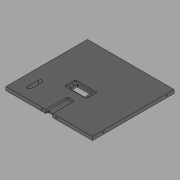
# Autodesk Inventor part: box_shelf
Saved by Autodesk Inventor 2019 (Build 230136000, 136)
## iProperties
Part Number: box_shelf
Material: Generic
Document SubType Name: Modeling
Designer: Javi
Appearance: Default
screws: 0,400 cm
Author: Javi
Autodesk Inventor part; units mm, degrees
ref_plane "YZ Plane" through (0, 0, 0) normal (1, 0, 0) x (0, 1, 0)
ref_plane "XZ Plane" through (0, 0, 0) normal (0, 1, 0) x (-1, 0, 0)
ref_plane "XY Plane" through (0, 0, 0) normal (0, 0, 1) x (1, 0, 0)
sketch "Sketch1" plane through (0, 0, 0) normal (0, 1, 0) x (-1, 0, 0)
  line L0 (0, 0) -> (-120, 0)
  line L1 (-120, 0) -> (-120, -226)
  line L2 (-120, -226) -> (0, -226)
  line L3 (0, -226) -> (0, 0)
  dimension "d0" = 120
  dimension "d1" = 226
  constraints: 8 end point, 2 parallel, 1 horizontal, 1 perpendicular
  measures "d0" distance of L2.end L1.end
  measures "d1" distance of L1.end L0.end
extrude "Extrusion1" add sketch "Sketch1" along normal blind 10
sketch "Sketch2" plane through (120, 0, 0) normal (1, 0, 0) x (0, 0, -1)
  circle A0 centre (30, 5) radius 2
  line L0 (0, 0) -> (0, 10) projected
  line L1 (0, 10) -> (226, 10) projected
  circle A1 centre (206, 5) radius 2
  dimension "d4" = 4
  dimension "d5" = 30
  dimension "d6" = 5
  dimension "d9" = 176
  constraints: 2 centre point, 1 horizontal, 2 other
  measures "d4" diameter of A0
  measures "d5" distance from line of L0 A0.centre
  measures "d6" distance from line of L1 A0.centre
  measures "d9" distance of A0.centre A1.centre
extrude "Extrusion2" cut sketch "Sketch2" against normal blind 10
sketch "Sketch3" plane through (0, 0, 0) normal (0, 0, 1) x (1, 0, 0)
  circle A0 centre (20, 5) radius 2
  line L0 (0, 10) -> (120, 10) projected
  line L1 (0, 0) -> (0, 10) projected
  dimension "d16" = 4
  dimension "d17" = 5
  dimension "d18" = 20
  constraints: 1 centre point
  measures "d16" diameter of A0
  measures "d17" distance from line of L0 A0.centre
  measures "d18" distance from line of L1 A0.centre
extrude "Extrusion3" cut sketch "Sketch3" against normal blind 10
mirror "Mirror1" about plane through (0, 0, -226) normal (-1, 0, 0)
sketch "Sketch4" plane through (0, 10, 0) normal (0, 1, 0) x (1, 0, 0)
  circle A0 centre (0, 97.45) radius 10
  line L0 (120, 0) -> (-120, 0) projected
  line L1 (-30.1, 107.45) -> (10.4, 107.45)
  line L2 (10.4, 107.45) -> (10.4, 87.45)
  line L3 (10.4, 87.45) -> (-30.1, 87.45)
  line L4 (-30.1, 87.45) -> (-30.1, 107.45)
  circle A1 centre (-34.65, 92.45) radius 1.75
  circle A2 centre (-34.65, 102.45) radius 1.75
  circle A3 centre (15.85, 92.45) radius 1.75
  circle A4 centre (15.85, 102.45) radius 1.75
  arc A5 (10.4, 107.45) -> (8.4, 107.45) centre (9.4, 107.45) ccw
  arc A6 (8.4, 87.45) -> (10.4, 87.45) centre (9.4, 87.45) ccw
  arc A7 (-28.1, 107.45) -> (-30.1, 107.45) centre (-29.1, 107.45) ccw
  arc A8 (-30.1, 87.45) -> (-28.1, 87.45) centre (-29.1, 87.45) ccw
  arc A9 (-90, 30) -> (-80, 30) centre (-85, 30) ccw
  arc A10 (-80, 60) -> (-90, 60) centre (-85, 60) ccw
  line L5 (-90, 30) -> (-90, 60)
  line L6 (-80, 30) -> (-80, 60)
  line L7 (-120, 0) -> (-120, 226) projected
  point P0 (0, 0)
  dimension "d21" = 97.45
  dimension "d22" = 0
  dimension "d23" = 20
  dimension "d24" = 20
  dimension "d27" = 10.4
  dimension "d28" = 3.5
  dimension "d31" = 10
  dimension "d34" = 50.5
  dimension "d37" = 5
  dimension "d38" = 4.55
  dimension "d39" = 30.1
  dimension "d50" = 1
  dimension "d54" = 10
  dimension "d55" = 30
  dimension "d56" = 30
  dimension "d57" = 30
  constraints: 12 end point, 12 point on circle, 11 centre point, 9 tangent, 4 equal radius, 4 point on line, 2 horizontal, 2 parallel, 2 perpendicular, 1 vertical, 6 other
  measures "d21" distance from line of L0 A0.centre
  measures "d22" horizontal distance of point (0, 0) A0.centre
  measures "d23" diameter of A0
  measures "d24" distance of L1.end L2.end
  measures "d27" distance from line of A0.centre L2
  measures "d28" diameter of A1
  measures "d31" distance of A1.centre A2.centre
  measures "d34" distance of A1.centre A3.centre
  measures "d37" distance from line of L3 A1.centre
  measures "d38" distance from line of L4 A1.centre
  measures "d39" distance from line of A0.centre L4
  measures "d50" radius of A5
  measures "d54" diameter of A10
  measures "d55" distance of L5.start L5.end
  measures "d56" distance between parallel lines of L7 L5
  measures "d57" distance from line of L0 A9.centre
extrude "Extrusion4" cut sketch "Sketch4" against normal through all
sketch "Sketch5" plane through (0, 10, 0) normal (0, 1, 0) x (1, 0, 0)
  line L0 (-37.1, 112.45) -> (17.4, 112.45)
  line L1 (20.4, 109.45) -> (20.4, 85.45)
  line L2 (17.4, 82.45) -> (-37.1, 82.45)
  line L3 (-40.1, 85.45) -> (-40.1, 109.45)
  line L4 (10.4, 107.45) -> (10.4, 87.45) projected
  line L5 (-28.1, 107.45) -> (8.4, 107.45) projected
  arc A0 (-40.1, 85.45) -> (-37.1, 82.45) centre (-37.1, 85.45) ccw
  arc A1 (-37.1, 112.45) -> (-40.1, 109.45) centre (-37.1, 109.45) ccw
  arc A2 (20.4, 109.45) -> (17.4, 112.45) centre (17.4, 109.45) ccw
  arc A3 (17.4, 82.45) -> (20.4, 85.45) centre (17.4, 85.45) ccw
  point P0 (0, 0)
  point P1 (-40.1, 112.45)
  point P2 (20.4, 82.45)
  point P3 (20.4, 112.45)
  point P4 (-40.1, 82.45)
  point P5 (-30.1, 107.45)
  dimension "d42" = 10
  dimension "d43" = 30
  dimension "d44" = 60.5
  dimension "d45" = 5
  dimension "d48" = 3
  constraints: 8 end point, 8 point on circle, 8 point on line, 8 tangent, 4 centre point, 3 equal radius, 2 parallel, 1 horizontal, 1 perpendicular
  measures "d42" distance between parallel lines of L1 L4
  measures "d43" distance of point (20.4, 112.45) point (20.4, 82.45)
  measures "d44" distance of point (20.4, 82.45) point (-40.1, 82.45)
  measures "d45" distance between parallel lines of L5 L0
  measures "d48" radius of A0
extrude "Extrusion5" cut sketch "Sketch5" against normal blind 4
sketch "Sketch6" plane through (0, 10, 0) normal (0, 1, 0) x (1, 0, 0)
  line L0 (-10, 0) -> (10, 0)
  line L1 (10, 0) -> (10, 57)
  line L2 (7, 60) -> (-7, 60)
  line L3 (-10, 57) -> (-10, 0)
  line L4 (120, 0) -> (-120, 0) projected
  arc A0 (-7, 60) -> (-10, 57) centre (-7, 57) ccw
  arc A1 (10, 57) -> (7, 60) centre (7, 57) ccw
  point P0 (0, 0)
  point P1 (10, 60)
  point P2 (-10, 60)
  dimension "d58" = 20
  dimension "d59" = 60
  dimension "d60" = 10
  dimension "d61" = 0
  dimension "d64" = 3
  constraints: 8 end point, 4 point on circle, 4 point on line, 4 tangent, 2 centre point, 2 parallel, 1 equal radius, 1 horizontal, 1 perpendicular
  measures "d58" distance of point (-10, 60) point (10, 60)
  measures "d59" distance of point (10, 60) L0.end
  measures "d60" distance from line of point (0, 0) L3
  measures "d61" distance between parallel lines of L4 L0
  measures "d64" radius of A0
extrude "Extrusion6" cut sketch "Sketch6" against normal blind 6
sketch "Sketch7" plane through (0, 4, 0) normal (0, 1, 0) x (1, 0, 0)
  line L0 (-10, 0) -> (-10, 57) projected
  line L1 (-10, 0) -> (10, 0)
  line L2 (10, 0) -> (10, 3)
  line L3 (7, 6) -> (-7, 6)
  line L4 (-10, 3) -> (-10, 0)
  arc A0 (-7, 6) -> (-10, 3) centre (-7, 3) ccw
  arc A1 (10, 3) -> (7, 6) centre (7, 3) ccw
  point P0 (0, 0)
  point P1 (10, 6)
  point P2 (-10, 6)
  dimension "d66" = 20
  dimension "d67" = 6
  dimension "d70" = 3
  constraints: 8 end point, 4 point on circle, 4 point on line, 4 tangent, 2 centre point, 2 parallel, 1 equal radius, 1 horizontal, 1 perpendicular
  measures "d66" distance of point (-10, 6) point (10, 6)
  measures "d67" distance of point (10, 6) L1.end
  measures "d70" radius of A0
extrude "Extrusion7" cut sketch "Sketch7" against normal through all
equation "\"d4\" = screws"
equation "\"d16\" = screws"
equation "\"screws\" = 4"
body "Solid1"
